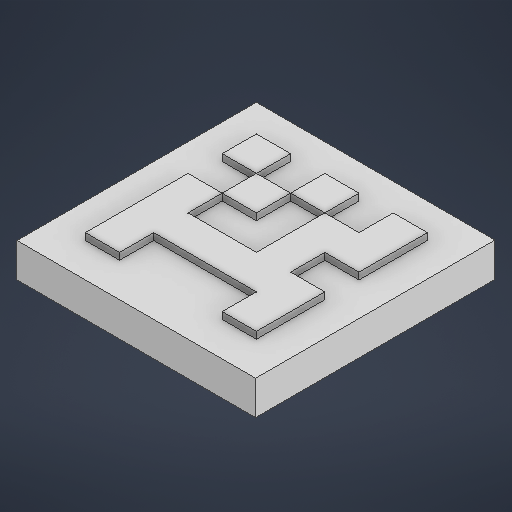
# Autodesk Inventor part: AprilTag
Saved by Autodesk Inventor 2026.1 (Build 301233000, 233)
## iProperties
Created: 2025-10-13
Part Number: AprilTag
Material: Generisch
Document SubType Name: Modeling
Designer: JurijLenz
Density: 1 g/cm^3
Appearance: Vorgabe
Author: JurijLenz
Autodesk Inventor part; units mm, degrees
ref_plane "YZ Plane" through (0, 0, 0) normal (1, 0, 0) x (0, 1, 0)
ref_plane "XZ Plane" through (0, 0, 0) normal (0, 1, 0) x (-1, 0, 0)
ref_plane "XY Plane" through (0, 0, 0) normal (0, 0, 1) x (1, 0, 0)
sketch "Skizze1" plane through (0, 0, 0) normal (0, 0, 1) x (1, 0, 0)
  line L0 (-7020.7506, -4267.5758) -> (-7020.7506, -4268.0775)
  line L1 (-7020.7506, -4268.0775) -> (-7020.2489, -4268.0775)
  line L2 (-7020.2489, -4268.0775) -> (-7019.7472, -4268.0775)
  line L3 (-7019.7472, -4268.0775) -> (-7019.7472, -4267.5758)
  line L4 (-7019.7472, -4267.5758) -> (-7019.7472, -4267.0742)
  line L5 (-7019.7472, -4267.0742) -> (-7019.2455, -4267.0742)
  line L6 (-7019.2455, -4267.0742) -> (-7018.7438, -4267.0742)
  line L7 (-7018.7438, -4267.0742) -> (-7018.7438, -4267.5758)
  line L8 (-7018.7438, -4267.5758) -> (-7018.7438, -4268.0775)
  line L9 (-7018.7438, -4268.0775) -> (-7018.2422, -4268.0775)
  line L10 (-7018.2422, -4268.0775) -> (-7017.7405, -4268.0775)
  line L11 (-7017.7405, -4268.0775) -> (-7017.7405, -4267.5758)
  line L12 (-7017.7405, -4267.5758) -> (-7017.7405, -4267.0742)
  line L13 (-7017.7405, -4267.0742) -> (-7017.2388, -4267.0742)
  line L14 (-7017.2388, -4267.0742) -> (-7016.7371, -4267.0742)
  line L15 (-7016.7371, -4267.0742) -> (-7016.7371, -4268.0775)
  line L16 (-7016.7371, -4268.0775) -> (-7016.7371, -4269.0809)
  line L17 (-7016.7371, -4269.0809) -> (-7017.2388, -4269.0809)
  line L18 (-7017.2388, -4269.0809) -> (-7017.7405, -4269.0809)
  line L19 (-7017.7405, -4269.0809) -> (-7017.7405, -4269.5826)
  line L20 (-7017.7405, -4269.5826) -> (-7017.7405, -4270.0843)
  line L21 (-7017.7405, -4270.0843) -> (-7017.2388, -4270.0843)
  line L22 (-7017.2388, -4270.0843) -> (-7016.7371, -4270.0843)
  line L23 (-7016.7371, -4270.0843) -> (-7016.7371, -4271.0876)
  line L24 (-7016.7371, -4271.0876) -> (-7016.7371, -4272.091)
  line L25 (-7016.7371, -4272.091) -> (-7017.2388, -4272.091)
  line L26 (-7017.2388, -4272.091) -> (-7017.7405, -4272.091)
  line L27 (-7017.7405, -4272.091) -> (-7017.7405, -4271.5893)
  line L28 (-7017.7405, -4271.5893) -> (-7017.7405, -4271.0876)
  line L29 (-7017.7405, -4271.0876) -> (-7019.2455, -4271.0876)
  line L30 (-7019.2455, -4271.0876) -> (-7020.7506, -4271.0876)
  line L31 (-7020.7506, -4271.0876) -> (-7020.7506, -4271.5893)
  line L32 (-7020.7506, -4271.5893) -> (-7020.7506, -4272.091)
  line L33 (-7020.7506, -4272.091) -> (-7021.2523, -4272.091)
  line L34 (-7021.2523, -4272.091) -> (-7021.7539, -4272.091)
  line L35 (-7021.7539, -4272.091) -> (-7021.7539, -4270.5859)
  line L36 (-7021.7539, -4270.5859) -> (-7021.7539, -4269.0809)
  line L37 (-7021.7539, -4269.0809) -> (-7021.2523, -4269.0809)
  line L38 (-7021.2523, -4269.0809) -> (-7020.7506, -4269.0809)
  line L39 (-7020.7506, -4269.0809) -> (-7020.7506, -4268.5792)
  line L40 (-7020.7506, -4268.5792) -> (-7020.7506, -4268.0775)
  line L41 (-7020.7506, -4268.0775) -> (-7021.2523, -4268.0775)
  line L42 (-7021.2523, -4268.0775) -> (-7021.7539, -4268.0775)
  line L43 (-7021.7539, -4268.0775) -> (-7021.7539, -4267.5758)
  line L44 (-7021.7539, -4267.5758) -> (-7021.7539, -4267.0742)
  line L45 (-7021.7539, -4267.0742) -> (-7021.2523, -4267.0742)
  line L46 (-7021.2523, -4267.0742) -> (-7020.7506, -4267.0742)
  line L47 (-7020.7506, -4267.0742) -> (-7020.7506, -4267.5758)
  line L48 (-7019.7472, -4268.5792) -> (-7019.7472, -4269.0809)
  line L49 (-7019.7472, -4269.0809) -> (-7020.2489, -4269.0809)
  line L50 (-7020.2489, -4269.0809) -> (-7020.7506, -4269.0809)
  line L51 (-7020.7506, -4269.0809) -> (-7020.7506, -4269.5826)
  line L52 (-7020.7506, -4269.5826) -> (-7020.7506, -4270.0843)
  line L53 (-7020.7506, -4270.0843) -> (-7019.7472, -4270.0843)
  line L54 (-7019.7472, -4270.0846) -> (-7018.7438, -4270.0846)
  line L55 (-7018.7438, -4270.0843) -> (-7018.7438, -4269.0809)
  line L56 (-7018.7438, -4269.0809) -> (-7018.7438, -4268.0775)
  line L57 (-7018.7438, -4268.0775) -> (-7019.2455, -4268.0775)
  line L58 (-7019.2455, -4268.0775) -> (-7019.7472, -4268.0775)
  line L59 (-7019.7472, -4268.0775) -> (-7019.7472, -4268.5792)
  line L60 (-7015.7576, -4266.0708) -> (-7022.7576, -4266.0708)
  line L61 (-7022.7576, -4266.0708) -> (-7022.7576, -4273.0944)
  line L62 (-7022.7576, -4273.0944) -> (-7015.7576, -4273.0944)
  line L63 (-7015.7576, -4273.0944) -> (-7015.7576, -4266.0708)
  dimension "d4" = 7
  dimension "d5" = 7.0236
  dimension "d6" = 1.0034
  dimension "d7" = 1.003
  dimension "d8" = 1.0034
  dimension "d9" = 1.0037
  constraints: 128 end point, 2 horizontal, 2 perpendicular
  measures "d4" distance of L60.start L60.end
  measures "d5" distance of L60.end L61.end
  measures "d6" distance between parallel lines of L60 L46
  measures "d7" distance between parallel lines of L54 L29
  measures "d8" distance between parallel lines of L62 L33
  measures "d9" distance between parallel lines of L61 L35
extrude "Extrusion1" add sketch "Skizze1" along normal blind 1 contours L58 L57 L56 L55 L54 L53 L52 L51 L50 L49 L48 L59 | L63 L62 L61 L60
extrude "Extrusion2" add sketch "Skizze1" along normal blind 1.2 contours L1 L2 L59 L48 L49 L50 L39 L40 | L0 L41 L42 L43 L44 L45 L46 L47 | L3 L4 L5 L6 L7 L8 L57 L58 | L51 L52 L53 L54 L55 L56 L9 L10 L11 L12 L13 L14 L15 L16 L17 L18 L19 L20 L21 L22 L23 L24 L25 L26 L27 L28 L29 L30 L31 L32 L33 L34 L35 L36 L37 L38
